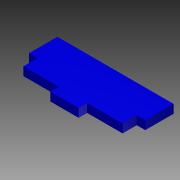
# Autodesk Inventor part: OpenROV 2.2 Dev Eboard ESC Seperator
Saved by Autodesk Inventor 2012 (Build 160160000, 160)
## iProperties
Created: 2012-01-08
Part Number: OpenROV 2.2 Dev Eboard ESC Seperator
Document SubType Name: Modeling
Designer: user
Density: 1 g/cm^3
Material: Default
Author: user
Autodesk Inventor part; units mm, degrees
ref_plane "YZ Plane" through (0, 0, 0) normal (1, 0, 0) x (0, 1, 0)
ref_plane "XZ Plane" through (0, 0, 0) normal (0, 1, 0) x (-1, 0, 0)
ref_plane "XY Plane" through (0, 0, 0) normal (0, 0, 1) x (1, 0, 0)
sketch "Sketch1" plane through (0, 0, 0) normal (0, 0, 1) x (1, 0, 0)
  line L0 (35, 0) -> (35, 5)
  line L1 (35, 15) -> (0, 15)
  line L2 (0, 5) -> (0, 0)
  line L3 (0, 15) -> (-3, 15)
  line L4 (-3, 15) -> (-3, 5)
  line L5 (-3, 5) -> (0, 5)
  line L6 (35, 15) -> (38, 15)
  line L7 (38, 15) -> (38, 5)
  line L8 (38, 5) -> (35, 5)
  line L9 (22.5, 0) -> (22.5, -3)
  line L10 (22.5, -3) -> (12.5, -3)
  line L11 (12.5, -3) -> (12.5, 0)
  line L12 (0, 0) -> (12.5, 0)
  line L13 (22.5, 0) -> (35, 0)
  dimension "d1" = 15
  dimension "d2" = 3
  dimension "d3" = 3
  dimension "d4" = 10
  dimension "d5" = 10
  dimension "d7" = 10
  dimension "d8" = 12.5
  dimension "d9" = 41
  dimension "d10" = 12.5
  dimension "d11" = 5
  dimension "d12" = 5
  dimension "d13" = 3
  constraints: 28 end point, 6 parallel, 4 horizontal, 4 perpendicular
  measures "d1" distance of L1.end L2.end
  measures "d2" distance of L4.end L2.start
  measures "d3" distance of L7.end L0.end
  measures "d4" distance of L6.end L7.end
  measures "d5" distance of L3.end L4.end
  measures "d7" distance of L9.end L10.end
  measures "d8" distance between parallel lines of L2 L11
  measures "d9" distance between parallel lines of L7 L4
  measures "d10" distance of L9.start L0.start
  measures "d11" distance of L0.start L0.end
  measures "d12" distance of L2.start L2.end
  measures "d13" distance of L9.start L9.end
extrude "Extrusion1" add sketch "Sketch1" along normal blind 3
body "Solid1"
